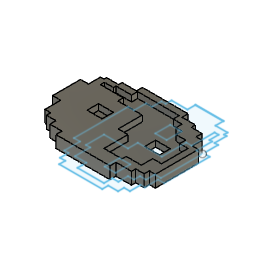
Yin-Yang-keychain (Autodesk Fusion 360 design; units mm, degrees)
Autodesk Fusion 360 part; units mm, degrees
sketch "Yin Yang" plane through (0, 0, 0) normal (0, 0, 1) x (1, 0, 0)
  line L0 (-23.2956, 29.4847) -> (0, 29.4847)
  line L1 (0, 29.4847) -> (0, 22.8951)
  line L2 (0, 22.8951) -> (10, 22.8951)
  line L3 (10, 22.8951) -> (10, 20)
  line L4 (10, 20) -> (12.1071, 20)
  line L5 (12.1071, 20) -> (12.1071, 10)
  line L6 (12.1071, 10) -> (15, 10)
  line L7 (15, 10) -> (15, -2.0318)
  line L8 (15, -2.0318) -> (20, -2.0318)
  line L9 (20, -2.0318) -> (20, -40)
  line L10 (20, -40) -> (15, -40)
  line L11 (15, -40) -> (15, -51.0886)
  line L12 (15, -51.0886) -> (11.6065, -51.0886)
  line L13 (11.6065, -51.0886) -> (11.6065, -60)
  line L14 (11.6065, -60) -> (6.745, -60)
  line L15 (6.745, -60) -> (6.745, -65)
  line L16 (6.745, -65) -> (-1.4301, -65)
  line L17 (-1.4301, -65) -> (-1.4301, -70)
  line L18 (-1.4301, -70) -> (-37.2472, -70)
  line L19 (-37.2472, -70) -> (-37.2472, -65)
  line L20 (-37.2472, -65) -> (-41.5428, -65)
  line L21 (-41.5428, -65) -> (-41.5428, -57.9737)
  line L22 (-41.5428, -57.9737) -> (-45, -57.9737)
  line L23 (-45, -57.9737) -> (-45, -45)
  line L24 (-45, -45) -> (-50, -45)
  line L25 (-50, -45) -> (-50, 0)
  line L26 (-50, 0) -> (-45, 0)
  line L27 (-45, 0) -> (-45, 10)
  line L28 (-45, 10) -> (-40, 10)
  line L29 (-40, 10) -> (-40, 17.848)
  line L30 (-40, 17.848) -> (-36.4664, 17.848)
  line L31 (-36.4664, 17.848) -> (-36.4664, 22.7525)
  line L32 (-36.4664, 22.7525) -> (-23.2956, 22.7525)
  line L33 (-23.2956, 22.7525) -> (-23.2956, 29.4847)
  line L34 (-19.4339, 4.603) -> (-11.8362, 4.603)
  line L35 (-11.8362, 4.603) -> (-10, 4.603)
  line L36 (-10, 4.603) -> (-10, -7.8294)
  line L37 (-10, -7.8294) -> (-19.4339, -7.8294)
  line L38 (-19.4339, -7.8294) -> (-19.4339, 4.603)
  line L39 (-16.5819, -40.5346) -> (-7.5822, -40.5346)
  line L40 (-7.5822, -40.5346) -> (-7.5822, -52.7983)
  line L41 (-7.5822, -52.7983) -> (-16.5819, -52.7983)
  line L42 (-16.5819, -52.7983) -> (-16.5819, -40.5346)
  line L43 (4.5405, 17.5451) -> (7.8452, 17.5451)
  line L44 (7.8452, 17.5451) -> (7.8452, 10)
  line L45 (7.8452, 10) -> (10, 10)
  line L46 (10, 10) -> (10, -3)
  line L47 (10, -3) -> (15, -3)
  line L48 (15, -2.0318) -> (15, -37.6367)
  line L49 (15, -37.6367) -> (10, -37.6367)
  line L50 (10, -37.6367) -> (10, -45)
  line L51 (10, -45) -> (5, -45)
  line L52 (5, -45) -> (5, -50)
  line L53 (5, -50) -> (0, -50)
  line L54 (0, -50) -> (0, -58.006)
  line L55 (0, -58.006) -> (-5, -58.006)
  line L56 (-5, -58.006) -> (-5, -65)
  line L57 (-5, -65) -> (-27.039, -65)
  line L58 (-27.039, -65) -> (-27.039, -61.1759)
  line L59 (-27.039, -61.1759) -> (-27.039, -57.6435)
  line L60 (-27.039, -57.6435) -> (-36.4761, -57.6435)
  line L61 (-36.4761, -57.6435) -> (-36.4761, -45)
  line L62 (-36.4761, -45) -> (-40, -45)
  line L63 (-40, -45) -> (-40, -30)
  line L64 (-40, -30) -> (-20, -30)
  line L65 (-20, -30) -> (-20, -21.8486)
  line L66 (-20, -21.8486) -> (0, -21.8486)
  line L67 (0, -21.8486) -> (0, -1.5133)
  line L68 (0, -1.5133) -> (4.5405, -1.5133)
  line L69 (4.5405, -1.5133) -> (4.5405, 17.5451)
  line L70 (-23.2956, 29.4847) -> (0, 29.4847)
  constraint horizontal L0
  constraint perpendicular L0 L1
  constraint perpendicular L1 L2
  constraint perpendicular L2 L3
  constraint perpendicular L3 L4
  constraint perpendicular L4 L5
  constraint perpendicular L5 L6
  constraint perpendicular L6 L7
  constraint perpendicular L7 L8
  constraint perpendicular L8 L9
  constraint perpendicular L9 L10
  constraint perpendicular L10 L11
  constraint perpendicular L11 L12
  constraint perpendicular L12 L13
  constraint perpendicular L13 L14
  constraint perpendicular L14 L15
  constraint perpendicular L15 L16
  constraint perpendicular L16 L17
  constraint perpendicular L17 L18
  constraint perpendicular L18 L19
  constraint perpendicular L19 L20
  constraint perpendicular L20 L21
  constraint perpendicular L21 L22
  constraint perpendicular L22 L23
  constraint perpendicular L23 L24
  constraint perpendicular L24 L25
  constraint perpendicular L25 L26
  constraint perpendicular L26 L27
  constraint perpendicular L27 L28
  constraint perpendicular L28 L29
  constraint perpendicular L29 L30
  constraint perpendicular L30 L31
  constraint perpendicular L31 L32
  constraint perpendicular L9 L34
  constraint perpendicular L9 L35
  constraint perpendicular L35 L36
  constraint perpendicular L36 L37
  constraint perpendicular L37 L38
  constraint horizontal L39
  constraint perpendicular L39 L40
  constraint perpendicular L40 L41
  constraint perpendicular L41 L42
  constraint perpendicular L5 L43
  constraint perpendicular L43 L44
  constraint perpendicular L44 L45
  constraint perpendicular L45 L46
  constraint perpendicular L46 L47
  constraint perpendicular L47 L48
  constraint perpendicular L48 L49
  constraint perpendicular L49 L50
  constraint perpendicular L50 L51
  constraint perpendicular L51 L52
  constraint perpendicular L52 L53
  constraint perpendicular L53 L54
  constraint perpendicular L54 L55
  constraint perpendicular L55 L56
  constraint perpendicular L54 L57
  constraint perpendicular L57 L58
  constraint perpendicular L57 L59
  constraint perpendicular L59 L60
  constraint perpendicular L60 L61
  constraint perpendicular L61 L62
  constraint perpendicular L60 L63
  constraint perpendicular L63 L64
  constraint perpendicular L64 L65
  constraint perpendicular L65 L66
  constraint perpendicular L66 L67
  constraint perpendicular L67 L68
  constraint perpendicular L68 L69
  constraint perpendicular L32 L33
extrude "Extrude2" add sketch "Yin Yang" along normal blind 10 contours L0 L1 L2 L3 L4 L5 L6 L7 L8 L9 L10 L11 L12 L13 L14 L15 L16 L17 L18 L19 L20 L21 L22 L23 L24 L25 L26 L27 L28 L29 L30 L31 L32 L33 L70
extrude "Extrude3" add sketch "Yin Yang" along normal blind 5 contours L34 L35 L36 L37 L38 | L43 L44 L45 L46 L47 L48 L49 L50 L51 L52 L53 L54 L55 L56 L57 L58 L59 L60 L61 L62 L63 L64 L65 L66 L67 L68 L69
move_body "Move1" bodies 1 to x (0, 1, 0) y (-1, 0, 0) z (0, 0, 1) at (-50, -10, 0)
named bodies: "Yin Yang"
